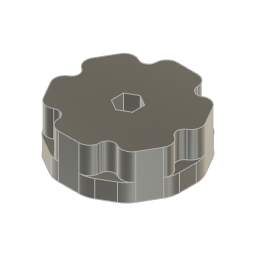
ogniwo-złożenie-v7 (Autodesk Fusion 360 archive; units mm, degrees)
design "zębatka"
Autodesk Fusion 360 part; units mm, degrees
sketch "Szkic1" plane through (0, 0, 0) normal (0, 0, 1) x (1, 0, 0)
  line L0 (0, 0) -> (16, 0)
  line L1 (16, 0) -> (24, 13.8564)
  line L2 (24, 13.8564) -> (16, 27.7128)
  line L3 (16, 27.7128) -> (0, 27.7128)
  line L4 (0, 27.7128) -> (-8, 13.8564)
  line L5 (-8, 13.8564) -> (0, 0)
  circle A0 centre (0, 0) radius 2.1
  circle A1 centre (16, 0) radius 2.1
  circle A2 centre (24, 13.8564) radius 2.1
  circle A3 centre (16, 27.7128) radius 2.1
  circle A4 centre (0, 27.7128) radius 2.1
  circle A5 centre (-8, 13.8564) radius 2.1
  circle A6 centre (8, 13.8564) radius 3
  line L6 (27.4641, 13.8564) -> (17.7321, 30.7128)
  line L7 (17.7321, 30.7128) -> (-1.7321, 30.7128)
  line L8 (-1.7321, 30.7128) -> (-11.4641, 13.8564)
  line L9 (-11.4641, 13.8564) -> (-1.7321, -3)
  line L10 (-1.7321, -3) -> (17.7321, -3)
  line L11 (17.7321, -3) -> (27.4641, 13.8564)
  line L12 (0, 0) -> (-1.7321, -3)
  line L13 (-1.8187, 1.05) -> (-3.5507, -1.95)
  line L14 (1.8187, -1.05) -> (0.0866, -4.05)
  line L15 (17.8187, 1.05) -> (19.5507, -1.95)
  line L16 (14.1813, -1.05) -> (15.9134, -4.05)
  line L17 (24, 15.9564) -> (27.4641, 15.9564)
  line L18 (24, 11.7564) -> (27.4641, 11.7564)
  line L19 (14.1813, 28.7628) -> (15.9134, 31.7628)
  line L20 (17.8187, 26.6628) -> (19.5507, 29.6628)
  line L21 (-1.8187, 26.6628) -> (-3.5507, 29.6628)
  line L22 (1.8187, 28.7628) -> (0.0866, 31.7628)
  line L23 (-8, 11.7564) -> (-11.4641, 11.7564)
  line L24 (-8, 15.9564) -> (-11.4641, 15.9564)
  line L25 (11, 15.5885) -> (8, 17.3205)
  line L26 (8, 17.3205) -> (5, 15.5885)
  line L27 (5, 15.5885) -> (5, 12.1244)
  line L28 (5, 12.1244) -> (8, 10.3923)
  line L29 (8, 10.3923) -> (11, 12.1244)
  line L30 (11, 12.1244) -> (11, 15.5885)
  point P0 (8, 13.8564)
  point P1 (8, 13.8564)
  dimension "d1" = 16
  dimension "d2" = 4.2
  dimension "d3" = 4.2
  dimension "d4" = 4.2
  dimension "d5" = 4.2
  dimension "d6" = 6
  dimension "d9" = 4.2
  dimension "d10" = 4.2
  dimension "d25" = 3
  dimension "d30" = 2.1
  dimension "d31" = -2.1
  dimension "d37" = 360
  constraint coincident L0.start L5.end
  constraint coincident L0.end L1.start
  constraint coincident L1.end L2.start
  constraint coincident L2.end L3.start
  constraint coincident L3.end L4.start
  constraint coincident L4.end L5.start
  constraint coincident P1 P0
  measures "d1" distance of L0.start L0.end
  measures "d2" diameter of A2
  measures "d3" diameter of A3
  measures "d4" diameter of A4
  measures "d5" diameter of A5
  measures "d6" diameter of A6
  measures "d9" diameter of A1
  measures "d10" diameter of A0
extrude "Wyciągnięcie proste1" add sketch "Szkic1" along normal blind 7.5 contours L0 L1 L2 L3 L4 L5 A0 A1 A2 A3 A4 A5 | A6 L29 L30 | A6 L25 L30 | A6 L25 L26 | A6 L28 L29 | A6 L26 L27 | A6 L27 L28
sketch "Szkic2" plane through (0, 0, 0) normal (0, 0, -1) x (1, 0, 0)
  circle A0 centre (8, -13.8564) radius 3
  line L0 (13.9, 0) -> (2.1, 0)
  arc A1 (-1.05, -1.8187) -> (2.1, 0) centre (0, 0) ccw
  line L1 (-1.05, -1.8187) -> (-6.95, -12.0378)
  arc A2 (-6.95, -15.6751) -> (-6.95, -12.0378) centre (-8, -13.8564) ccw
  line L2 (-6.95, -15.6751) -> (-1.05, -25.8942)
  arc A3 (2.1, -27.7128) -> (-1.05, -25.8942) centre (0, -27.7128) ccw
  line L3 (2.1, -27.7128) -> (13.9, -27.7128)
  arc A4 (17.05, -25.8942) -> (13.9, -27.7128) centre (16, -27.7128) ccw
  line L4 (17.05, -25.8942) -> (22.95, -15.6751)
  arc A5 (22.95, -12.0378) -> (22.95, -15.6751) centre (24, -13.8564) ccw
  line L5 (22.95, -12.0378) -> (17.05, -1.8187)
  arc A6 (13.9, 0) -> (17.05, -1.8187) centre (16, 0) ccw
  line L6 (8, -13.8564) -> (0, 0)
  line L7 (0, 0) -> (-1.4, 2.4249)
  line L8 (0, 0) -> (-0.5, 0.866)
  line L9 (-0.5, 0.866) -> (2.2, 2.4249)
  line L10 (-0.5, 0.866) -> (-3.2, -0.6928)
  line L11 (16, 0) -> (17.4, 2.4249)
  line L12 (16, 0) -> (16.5, 0.866)
  line L13 (16.5, 0.866) -> (19.2, -0.6928)
  line L14 (16.5, 0.866) -> (13.8, 2.4249)
  line L15 (24, -13.8564) -> (26.8, -13.8564)
  line L16 (24, -13.8564) -> (25, -13.8564)
  line L17 (25, -13.8564) -> (25, -16.9741)
  line L18 (25, -13.8564) -> (25, -10.7387)
  line L19 (16, -27.7128) -> (17.4, -30.1377)
  line L20 (16, -27.7128) -> (16.5, -28.5788)
  line L21 (16.5, -28.5788) -> (13.8, -30.1377)
  line L22 (16.5, -28.5788) -> (19.2, -27.02)
  line L23 (0, -27.7128) -> (-1.4, -30.1377)
  line L24 (0, -27.7128) -> (-0.5, -28.5788)
  line L25 (-0.5, -28.5788) -> (2.2, -30.1377)
  line L26 (-0.5, -28.5788) -> (-3.2, -27.02)
  line L27 (-8, -13.8564) -> (-10.8, -13.8564)
  line L28 (-8, -13.8564) -> (-9, -13.8564)
  line L29 (-9, -13.8564) -> (-9, -16.9741)
  line L30 (-9, -13.8564) -> (-9, -10.7387)
  line L31 (19.2, -27.02) -> (21.7535, -25.5457)
  line L32 (21.7535, -25.5457) -> (12.0533, -31.1462)
  line L33 (25, -10.7387) -> (25, -7)
  line L34 (25, -7) -> (25, -16.9741)
  line L35 (25, -21.3448) -> (25, -16.5)
  line L36 (13.8, 2.4249) -> (11.1881, 3.9329)
  line L37 (11.1881, 3.9329) -> (22.533, -2.6171)
  line L38 (2.2, 2.4249) -> (5.8269, 4.5189)
  line L39 (5.8269, 4.5189) -> (-6.533, -2.6171)
  line L40 (-9, -16.9741) -> (-9, -24)
  line L41 (-9, -24) -> (-9, -7)
  line L42 (-3.2, -27.02) -> (-8.2097, -24.1276)
  line L43 (-8.2097, -24.1276) -> (5.8633, -32.2527)
  arc A7 (13.9, -30.7128) -> (16.6679, -28.8697) centre (13.9, -27.7128) ccw
  line L44 (2.1, -30.7128) -> (13.9, -30.7128)
  arc A8 (-0.6679, -28.8697) -> (2.1, -30.7128) centre (2.1, -27.7128) ccw
  arc A9 (-3.6481, -27.3942) -> (-0.6679, -28.8697) centre (-1.05, -25.8942) ccw
  line L45 (-9.5481, -17.1751) -> (-3.6481, -27.3942)
  arc A10 (-9.3359, -13.8564) -> (-9.5481, -17.1751) centre (-6.95, -15.6751) ccw
  arc A11 (-9.5481, -10.5378) -> (-9.3359, -13.8564) centre (-6.95, -12.0378) ccw
  line L46 (-3.6481, -0.3187) -> (-9.5481, -10.5378)
  arc A12 (-0.6679, 1.1569) -> (-3.6481, -0.3187) centre (-1.05, -1.8187) ccw
  arc A13 (2.1, 3) -> (-0.6679, 1.1569) centre (2.1, 0) ccw
  line L47 (13.9, 3) -> (2.1, 3)
  arc A14 (16.6679, 1.1569) -> (13.9, 3) centre (13.9, 0) ccw
  arc A15 (19.6481, -0.3187) -> (16.6679, 1.1569) centre (17.05, -1.8187) ccw
  line L48 (25.5481, -10.5378) -> (19.6481, -0.3187)
  arc A16 (25.3359, -13.8564) -> (25.5481, -10.5378) centre (22.95, -12.0378) ccw
  arc A17 (25.5481, -17.1751) -> (25.3359, -13.8564) centre (22.95, -15.6751) ccw
  line L49 (19.6481, -27.3942) -> (25.5481, -17.1751)
  arc A18 (16.6679, -28.8697) -> (19.6481, -27.3942) centre (17.05, -25.8942) ccw
  point P0 (8, -13.8564)
  dimension "d11" = 2.8
  dimension "d14" = 1
  dimension "d15" = 1
  dimension "d16" = 1
  dimension "d17" = 1
  dimension "d18" = 1
  dimension "d19" = 1
  dimension "d40" = 3
  constraint coincident P0 A0.centre
  constraint coincident A1.centre L6.end
  constraint parallel L6 L7
  constraint parallel L7 L8
  constraint perpendicular L7 L9
  constraint perpendicular L7 L10
  constraint coincident A6.centre L11.start
  constraint parallel L11 L12
  constraint perpendicular L12 L13
  constraint perpendicular L11 L14
  constraint coincident A5.centre L15.start
  constraint parallel L15 L16
  constraint perpendicular L15 L17
  constraint perpendicular L15 L18
  constraint coincident A4.centre L19.start
  constraint parallel L19 L20
  constraint perpendicular L20 L21
  constraint perpendicular L19 L22
  constraint coincident A3.centre L23.start
  constraint parallel L23 L24
  constraint perpendicular L23 L25
  constraint perpendicular L24 L26
  constraint coincident A2.centre L27.start
  constraint parallel L27 L28
  constraint perpendicular L28 L29
  constraint perpendicular L27 L30
  constraint parallel L22 L31
  constraint parallel L21 L32
  constraint parallel L18 L33
  constraint perpendicular L16 L34
  constraint coincident L34 L35.end
  constraint parallel L34 L35
  constraint parallel L14 L36
  constraint perpendicular L11 L37
  constraint parallel L9 L38
  constraint perpendicular L7 L39
  constraint parallel L29 L40
  constraint perpendicular L28 L41
  constraint parallel L26 L42
  constraint parallel L42 L43
  measures "d11" distance of A1.centre L7.end
  measures "d14" distance of A1.centre L8.end
  measures "d15" distance of A6.centre L12.end
  measures "d16" distance of A5.centre L16.end
  measures "d17" distance of A4.centre L20.end
  measures "d18" distance of A3.centre L24.end
  measures "d19" distance of A2.centre L28.end
  measures "d40" distance of L3.end
extrude "Wyciągnięcie proste2" add sketch "Szkic2" along normal blind 5 contours A0 | L0 A1 L1 A2 L2 A3 L3 A4 L4 A5 L5 A6
extrude "Wyciągnięcie proste3" add sketch "Szkic2" along normal blind 5 contours L9 L10 L13 L14 L17 L18 L21 L22 L25 L26 L29 L30 L31 L32 L33 L34 L35 L36 L37 L38 L39 L40 L41 L42 L43 L44 L45 L46 L47 L48 L49
extrude "Wyciągnięcie proste4" add sketch "Szkic2" along normal blind 5 contours L9 L10 L13 L14 L17 L18 L21 L22 L25 L26 L29 L30 L31 L32 L33 L34 L35 L36 L37 L38 L39 L40 L41 L42 L43 L44 L45 L46 L47 L48 L49
extrude "Wyciągnięcie proste5" add sketch "Szkic1" along normal blind 7.5 contours L0 A0 A1 L10 L14 L16 | L5 A0 A5 L9 L13 L23 | L1 A1 A2 L11 L15 L18 | L4 A4 A5 L8 L21 L24 | L2 A2 A3 L6 L17 L20 | L3 A3 A4 L7 L19 L22
fillet "Zaokrąglenie3" radius 3 12 edges at (0.6928, -3, 3.75) (15.3072, -3, 3.75) (26.2517, 11.7564, 3.75) (26.2517, 15.9564, 3.75) (18.9445, 28.6128, 3.75) (15.3072, 30.7128, 3.75) (0.6928, 30.7128, 3.75) (-2.9445, 28.6128, 3.75) (-10.2517, 15.9564, 3.75) (-10.2517, 11.7564, 3.75) (-2.9445, -0.9, 3.75) (18.9445, -0.9, 3.75)
fillet "Zaokrąglenie4" radius 7.083 12 edges at (3.1962, -3, -2.5) (12.8038, -3, -2.5) (20.1962, 1.2679, -2.5) (25, 9.5885, -2.5) (25, 18.1244, -2.5) (20.1962, 26.4449, -2.5) (12.8038, 30.7128, -2.5) (3.1962, 30.7128, -2.5) (-4.1962, 26.4449, -2.5) (-9, 18.1244, -2.5) (-9, 9.5885, -2.5) (-4.1962, 1.2679, -2.5)
extrude "Wyciągnięcie proste7" cut sketch "Szkic1" 1 faces at (8.8808, 14.5589, 0) along normal mid plane 38 contours A6 L29 L30 | A6 L25 L30 | A6 L25 L26 | A6 L28 L29 | A6 L26 L27 | A6 L27 L28

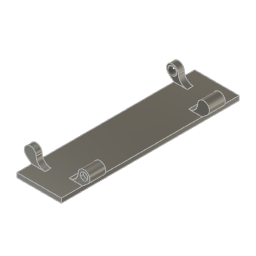
design "ogniwo prototyp"
Autodesk Fusion 360 part; units mm, degrees
sketch "Szkic1" plane through (0, 0, 0) normal (0, 0, 1) x (1, 0, 0)
  line L0 (0, 0) -> (15, 0)
  line L1 (15, 0) -> (15, 60)
  line L2 (15, 60) -> (0, 60)
  line L3 (0, 60) -> (0, 0)
  dimension "d1" = 15
  dimension "d2" = 60
  constraint horizontal L0
  constraint vertical L1
  constraint horizontal L2
  constraint vertical L3
  constraint coincident L0.start L3.end
  measures "d1" distance of L0.start L0.end
  measures "d2" distance of L0.start L2.end
extrude "Wyciągnięcie proste1" add sketch "Szkic1" along normal blind 1.5
sketch "Szkic2" plane through (0, 0, 0) normal (0, -1, 0) x (1, 0, 0)
  line L0 (0, 0) -> (15, 0)
  line L1 (15, 0) -> (15, 1.5)
  line L2 (15, 1.5) -> (0, 1.5)
  line L3 (0, 1.5) -> (0, 0)
  circle A0 centre (-0.5018, 4.5) radius 1.5
  circle A1 centre (-0.5018, 4.5) radius 2
  line L4 (0, 1.5) -> (-1.7711, 2.9544)
  line L5 (-0.5018, 4.5) -> (0.9124, 5.9142)
  line L6 (-0.5018, 4.5) -> (2, 4.5) construction
  line L7 (2, 4.5) -> (2, 4.5)
  line L8 (5, 1.5) -> (5, 1.5)
  line L9 (1.4982, 4.5) -> (1.4982, 4.5)
  line L10 (4.4982, 1.5) -> (4.4982, 1.5)
  arc A2 (1.4982, 4.5) -> (4.4982, 1.5) centre (4.4982, 4.5) ccw
  point P0 (2, 1.5)
  point P1 (1.4982, 1.5)
  dimension "d5" = 45
  dimension "d6" = 3
  dimension "d18" = 3
  dimension "d19" = 3
  constraint coincident L2.end L3.start
  constraint concentric A0 A1
  constraint coincident A1 L4.end
  constraint tangent A1 L4
  constraint horizontal L6
  constraint coincident A0.centre A1.centre
  constraint coincident A1 L5.end
  constraint coincident L2 P0
  constraint coincident P0 L7
  constraint coincident P0 L8
  constraint coincident A1 L9.start
  constraint coincident L6 L9.start
  constraint coincident L2 P1
  constraint coincident P1 L9
  constraint coincident P1 L10
  measures "d5" angle of L5 L6
  measures "d6" distance of P0 L8.start
  measures "d18" distance of P1 L10.start
  measures "d19" radius of A2
extrude "Wyciągnięcie proste2" add sketch "Szkic2" against normal blind 2 from surface at -5 contours L2 A1 L4 A2 | A1 | A0
sketch "Szkic3" plane through (0, 7, 0) normal (0, 1, 0) x (-1, 0, 0)
  arc A0 (1.7711, 2.9544) -> (-1.4982, 4.5) centre (0.5018, 4.5) ccw
  line L0 (-4.4982, 1.5) -> (0, 1.5)
  line L1 (0, 1.5) -> (1.7711, 2.9544)
  circle A1 centre (0.5018, 4.5) radius 1.5
  line L2 (0.5018, 4.5) -> (2.0018, 4.5)
  arc A2 (-4.4982, 1.5) -> (-1.4982, 4.5) centre (-4.4982, 4.5) ccw
  dimension "d11" = 3
  constraint concentric A0 A1
  constraint coincident A0.centre A1.centre
  constraint coincident A1 L2.end
  constraint horizontal L2
  measures "d11" diameter of A1
sketch "Szkic5" plane through (0, 0, 4.5) normal (0, 0, -1) x (1, 0, 0)
  line L0 (-0.5018, -7) -> (-2.0018, -7)
  line L1 (-2.0018, -7) -> (-2.0018, -8)
  line L2 (-2.0018, -8) -> (-0.5018, -8)
  line L3 (-0.5018, -8) -> (-0.5018, -7)
  line L4 (-2.0018, -7) -> (1, -7)
  arc A0 (-2.0018, -7) -> (1, -7) centre (-0.5009, -6.3736) ccw
  constraint coincident L0.end L1.start
  constraint perpendicular L3 L4
  constraint coincident L2.end A0
revolve "Obrót2" add sketch "Szkic5" angle 360 about axis through (-0.5018, 8, 4.5) along (0, -1, 0) contours L0 L3 L4 A0
sketch "Szkic6" plane through (0, 0, 0) normal (0, -1, 0) x (1, 0, 0)
  circle A0 centre (15.5, 4.5) radius 1.3
  circle A1 centre (15.5, 4.5) radius 2
  line L0 (15, 1.5) -> (16.77, 2.955)
  line L1 (13.5, 4.5) -> (13.5, 4.5)
  line L2 (10.5, 1.5) -> (10, 1.5)
  line L3 (13.5, 1.5) -> (15, 1.5)
  arc A2 (10.5, 1.5) -> (13.5, 4.5) centre (10.5, 4.5) ccw
  line L4 (10, 1.5) -> (10.1, 1.5)
  line L5 (13.5, 1.5) -> (10.25, 1.5)
  dimension "d26" = 2.6
  dimension "d27" = 3
  constraint coincident A1 L0.end
  constraint tangent A1 L0
  constraint coincident A1 L1.start
  constraint coincident L3.start L1
  constraint coincident L3.start L2
  constraint tangent L2 A2
  constraint coincident L2 L4.end
  constraint midpoint L2 L5.end
  constraint parallel L2 L5
  measures "d26" diameter of A0
  measures "d27" radius of A2
extrude "Wyciągnięcie proste7" add sketch "Szkic6" against normal blind 5 from surface at -7.5 contours A0 | A1 | A1 L0 L3 A2 L5
sketch "Szkic7" plane through (0, 7.5, 0) normal (0, -1, 0) x (1, 0, 0)
  line L0 (15, 1.5) -> (16.77, 2.955)
  arc A0 (16.77, 2.955) -> (13.5, 4.5) centre (15.5, 4.5) ccw
  arc A1 (10.5, 1.5) -> (13.5, 4.5) centre (10.5, 4.5) ccw
  line L1 (10.5, 1.5) -> (15, 1.5)
  circle A2 centre (15.5, 4.5) radius 1.25
  dimension "d31" = 2.5
  constraint concentric A0 A2
  measures "d31" diameter of A2
extrude "Wyciągnięcie proste8" cut sketch "Szkic7" against normal blind 0.6 contours A2
extrude "Wyciągnięcie proste9" add sketch "Szkic2" along normal blind 2 from surface at -55 contours L2 A1 L4 A2 | A1 | A0
sketch "Szkic8" plane through (0, 53, 0) normal (0, -1, 0) x (1, 0, 0)
  arc A0 (1.4982, 4.5) -> (-1.7711, 2.9544) centre (-0.5018, 4.5) ccw
  line L0 (-1.7711, 2.9544) -> (0, 1.5)
  line L1 (0, 1.5) -> (4.4982, 1.5)
  arc A1 (1.4982, 4.5) -> (4.4982, 1.5) centre (4.4982, 4.5) ccw
  circle A2 centre (-0.5018, 4.5) radius 1.5
  line L2 (-0.5018, 4.5) -> (-2.0018, 4.5)
  dimension "d37" = 3
  constraint concentric A0 A2
  constraint coincident A0.centre A2.centre
  constraint coincident A2 L2.end
  constraint horizontal L2
  measures "d37" diameter of A2
sketch "Szkic9" plane through (0, 0, 4.5) normal (0, 0, 1) x (-1, 0, 0)
  line L0 (0.5018, -53) -> (2.0018, -53)
  line L1 (2.0018, -53) -> (2.0018, -52)
  line L2 (2.0018, -52) -> (0.5018, -52)
  line L3 (0.5018, -52) -> (0.5018, -53)
  line L4 (2.0018, -53) -> (-0.9982, -53)
  arc A0 (2.0018, -53) -> (-0.9982, -53) centre (0.5018, -53.625) ccw
  dimension "d40" = 3
  constraint coincident L0.end L1.start
  constraint perpendicular L1 L4
  constraint coincident L2.end A0
  measures "d40" distance of L0.end L4.end
revolve "Obrót3" add sketch "Szkic9" angle 360 about axis through (-0.5018, 52, 4.5) along (0, 1, 0) contours L0 L3 L4 A0
extrude "Wyciągnięcie proste11" add sketch "Szkic6" along normal blind 5 from surface at -52.5 contours A0 | A1 | A1 L0 L3 A2 L5
sketch "Szkic10" plane through (0, 52.5, 0) normal (0, 1, 0) x (-1, 0, 0)
  line L0 (-16.77, 2.955) -> (-15, 1.5)
  line L1 (-15, 1.5) -> (-10.5, 1.5)
  arc A0 (-13.5, 4.5) -> (-10.5, 1.5) centre (-10.5, 4.5) ccw
  arc A1 (-13.5, 4.5) -> (-16.77, 2.955) centre (-15.5, 4.5) ccw
  circle A2 centre (-15.5, 4.5) radius 1.25
  dimension "d45" = 2.5
  constraint concentric A1 A2
  measures "d45" diameter of A2
extrude "Wyciągnięcie proste12" cut sketch "Szkic10" against normal blind 0.6 contours A2
extrude "Wyciągnięcie proste13" add 1 faces at (14.4583, 7.5, 2.1392) along direction (0, -1, 0) blind 0.35
extrude "Wyciągnięcie proste14" add sketch "Szkic10" along normal blind 0.35
